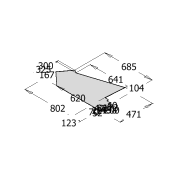
# Autodesk Inventor part: Contracted_profile
Saved by Autodesk Inventor 2022 (Build 260153000, 153)
## iProperties
Created: 2022-10-05
Part Number: Contracted_profile
Material: Generic
Document SubType Name: Modeling
Designer: dell
Mass: 254.845 g
Surface Area: 5120.54 cm^2
Volume: 254.845 cm^3
Density: 1 g/cm^3
Appearance: Default
Author: dell
Autodesk Inventor part; units mm, degrees
ref_plane "YZ Plane" through (0, 0, 0) normal (1, 0, 0) x (0, 1, 0)
ref_plane "XZ Plane" through (0, 0, 0) normal (0, 1, 0) x (-1, 0, 0)
ref_plane "XY Plane" through (0, 0, 0) normal (0, 0, 1) x (1, 0, 0)
sketch "Sketch1" plane through (0, 0, 0) normal (0, 1, 0) x (-1, 0, 0)
  line L0 (0, 0) -> (620, 0)
  line L1 (620, 0) -> (802, -167)
  line L2 (802, -167) -> (685, -325)
  line L3 (685, -325) -> (641, -300)
  line L4 (641, -300) -> (104, -471)
  line L5 (104, -471) -> (123, -200)
  line L6 (123, -200) -> (70, -198)
  line L7 (70, -198) -> (70, -173)
  line L8 (70, -173) -> (22, -173)
  line L9 (22, -173) -> (22, -143)
  line L10 (22, -143) -> (-40, -143)
  line L11 (-40, -143) -> (-52, -80)
  line L12 (-52, -80) -> (-52, -42)
  line L13 (0, 0) -> (0, -42)
  line L14 (0, -42) -> (-52, -42)
  dimension "d0" = 620
  dimension "d1" = 802
  dimension "d2" = 167
  dimension "d3" = 685
  dimension "d4" = 325
  dimension "d5" = 641
  dimension "d6" = 300
  dimension "d7" = 104
  dimension "d8" = 471
  dimension "d9" = 123
  dimension "d10" = 200
  dimension "d11" = 70
  dimension "d12" = 198
  dimension "d13" = 173
  dimension "d14" = 22
  dimension "d15" = 143
  dimension "d16" = 40
  dimension "d17" = 80
  dimension "d18" = 52
  dimension "d19" = 42
  constraints: 30 end point, 4 vertical, 3 horizontal, 1 perpendicular
  measures "d0" distance of L0.start L0.end
  measures "d1" horizontal distance of L0.start L1.end
  measures "d2" vertical distance of L0.end L1.end
  measures "d3" horizontal distance of L0.start L2.end
  measures "d4" vertical distance of L0.start L2.end
  measures "d5" horizontal distance of L0.start L3.end
  measures "d6" vertical distance of L0.start L3.end
  measures "d7" horizontal distance of L0.start L4.end
  measures "d8" vertical distance of L0.start L4.end
  measures "d9" horizontal distance of L0.start L5.end
  measures "d10" vertical distance of L0.start L5.end
  measures "d11" horizontal distance of L0.start L6.end
  measures "d12" vertical distance of L0.start L6.end
  measures "d13" vertical distance of L0.start L7.end
  measures "d14" horizontal distance of L0.start L8.end
  measures "d15" vertical distance of L0.start L9.end
  measures "d16" horizontal distance of L0.start L10.end
  measures "d17" vertical distance of L0.start L11.end
  measures "d18" horizontal distance of L0.start L11.end
  measures "d19" vertical distance of L0.start L12.end
extrude "Extrusion1" add sketch "Sketch1" along normal blind 1
body "Solid1"
